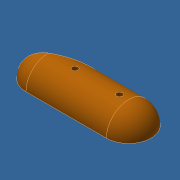
# Autodesk Inventor part: P1704_002
Saved by Autodesk Inventor 2019 (Build 230136000, 136)
## iProperties
Created: 2019-05-02
Part Number: P1704_002
Project: P1704 Manette
Material: PLA
Description: Main droite intérieur
Document SubType Name: Modeling
Designer: Joan.MAILLARD
Authority: brut Ø
Density: 1.25 g/cm^3
Appearance: Orange
Material number: ---
Author: Joan.MAILLARD
Title: P1704_002_mainDroiteInterieur
Autodesk Inventor part; units mm, degrees
ref_plane "Plan YZ" through (0, 0, 0) normal (1, 0, 0) x (0, 1, 0)
ref_plane "Plan XZ" through (0, 0, 0) normal (0, 1, 0) x (-1, 0, 0)
ref_plane "Plan XY" through (0, 0, 0) normal (0, 0, 1) x (1, 0, 0)
sketch "Esquisse1" plane through (0, 0, 0) normal (0, 0, 1) x (1, 0, 0)
  arc A0 (25, 25) -> (0, 0) centre (25, 0) ccw
  line L0 (25, 25) -> (115, 25)
  arc A1 (140, 0) -> (115, 25) centre (115, 0) ccw
  line L1 (0, 0) -> (132.1239, 0) construction
  line L2 (0, 0) -> (140, 0)
  dimension "d0" = 25
  dimension "d1" = 90
  constraints: 6 end point, 4 point on circle, 3 horizontal, 3 point on line, 2 centre point, 1 equal radius, 1 tangent
  measures "d0" distance between parallel lines of L1 L0
  measures "d1" distance of L0.start L0.end
revolve "Révolution1" add sketch "Esquisse1" angle 180 about axis through (0, 0, 0) along (1, 0, 0)
sketch "Esquisse6" plane through (115, 25, 0) normal (0, 0, -1) x (-1, 0, 0)
  line L0 (90, -25) -> (111.6506, -37.5)
  line L1 (111.6506, -37.5) -> (124.1506, -15.8494)
  line L2 (124.1506, -15.8494) -> (59.1987, 21.6506)
  line L3 (59.1987, 21.6506) -> (46.6987, 0)
  line L4 (46.6987, 0) -> (90, -25)
  arc A0 (90, -50) -> (90, 0) centre (90, -25) ccw projected
  line L5 (90, 0) -> (0, 0) projected
  line L6 (115, -25) -> (-35.1202, -25) construction
  dimension "d3" = 150
  constraints: 12 end point, 3 perpendicular, 1 coincident, 1 collinear, 1 horizontal, 1 point on circle, 1 point on line, 1 tangent
  measures "d3" angle of L6 L0
extrude "Extrusion1" cut sketch "Esquisse6" against normal blind 25 contours L4 L5 A0 L0
ref_plane "Plan de construction1" through (115, -25, 25) normal (0, 0, -1) x (-1, 0, 0)
sketch "Esquisse7" plane through (115, -25, 25) normal (0, 0, -1) x (-1, 0, 0)
  circle A0 centre (10, 25) radius 1.7
  circle A1 centre (60, 25) radius 1.7
  line L0 (0, 50) -> (0, 0) projected
  line L1 (10, 25) -> (10, 0) construction
  line L2 (10, 25) -> (10, 50) construction
  line L3 (60, 25) -> (60, 0) construction
  line L4 (60, 25) -> (60, 50) construction
  line L5 (0, 50) -> (95.4771, 50) construction
  line L6 (0, 0) -> (90, 0) construction
  point P0 (115, 25)
  dimension "d7" = 10
  dimension "d8" = 50
  dimension "d9" = 3.4
  dimension "d10" = 3.4
  constraints: 10 end point, 4 point on line, 4 vertical, 2 centre point, 2 collinear, 1 horizontal
  measures "d7" distance from line of L0 L1.start
  measures "d8" distance of L1.start L3.start
  measures "d9" diameter of A0
  measures "d10" diameter of A1
extrude "Extrusion2" cut sketch "Esquisse7" along normal blind 25
sketch "Esquisse8" plane through (115, -25, 25) normal (0, 0, -1) x (-1, 0, 0)
  circle A0 centre (10, 25) radius 3.25
  circle A1 centre (60, 25) radius 3.25
  circle A2 centre (10, 25) radius 1.7 projected
  circle A3 centre (60, 25) radius 1.7 projected
  point P0 (115, 25)
  dimension "d13" = 6.5
  dimension "d14" = 6.5
  constraints: 2 centre point, 2 concentric
  measures "d13" diameter of A0
  measures "d14" diameter of A1
extrude "Extrusion3" cut sketch "Esquisse8" along normal blind 12 contours A0 | A1 | A2 | A3
equation "\"d10\" = d9"
equation "\"d14\" = d13"
